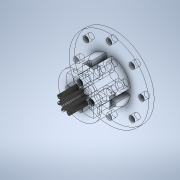
# Autodesk Inventor part: fixation_circle
Saved by Autodesk Inventor 2022.3 (Build 263350000, 350)
## iProperties
Created: 2022-01-31
Part Number: fixation_circle
Material: Generic
Document SubType Name: Modeling
Designer: Martijn
Density: 1 g/cm^3
Appearance: Default
Author: Martijn
Autodesk Inventor part; units mm, degrees
(part 1 of 2)
ref_plane "YZ Plane" through (0, 0, 0) normal (1, 0, 0) x (0, 1, 0)
ref_plane "XZ Plane" through (0, 0, 0) normal (0, 1, 0) x (-1, 0, 0)
ref_plane "XY Plane" through (0, 0, 0) normal (0, 0, 1) x (1, 0, 0)
sketch "Sketch1" plane through (0, 0, 0) normal (0, 0, 1) x (1, 0, 0)
  circle A0 centre (0, 0) radius 22
  circle A1 centre (0, 0) radius 2.6
  line L0 (-30.8, 0) -> (30.8, 0) projected
  line L1 (0, -30.8) -> (0, 30.8) projected
  dimension "d0" = 44
  dimension "d3" = 5.2
  dimension "d21" = 0
  constraints: 2 centre point, 2 coincident, 1 midpoint
  measures "d0" diameter of A0
  measures "d3" diameter of A1
  measures "d21" distance from line of L1 point (0, 0)
extrude "Extrusion1" add sketch "Sketch1" along normal blind 3 contours L0 A1 L1 A0 | A0 L1 A1 L0 | L1 A1 L0 A0 | A0 L0 A1 L1
sketch "Sketch3" plane through (0, 0, 3) normal (0, 0, 1) x (1, 0, 0)
  circle A0 centre (-18, 0) radius 1.6
  circle A1 centre (0, 0) radius 2.6 projected
  line L0 (-18, 0) -> (0, 0)
  line L1 (-63.2, 0) -> (36.2, 0) projected
  dimension "d11" = 3.2
  dimension "d12" = 18
  constraints: 2 end point, 1 centre point, 1 collinear
  measures "d11" diameter of A0
  measures "d12" distance of L0.end L0.start
extrude "Extrusion3" cut sketch "Sketch3" against normal blind 3 contours L0 L1 A0 | A0 L1 L0
pattern_circular "Circular Pattern2" count 8 over 360 about axis through (0, 0, 0) along (0, 0, 1) of "Extrusion3"
sketch "Sketch4" plane through (0, 0, 3) normal (0, 0, 1) x (1, 0, 0)
  circle A0 centre (0, 0) radius 12
  circle A1 centre (0, 0) radius 22 projected
  dimension "d20" = 24
  constraints: 1 centre point, 1 coincident, 1 concentric
  measures "d20" diameter of A0
extrude "Extrusion4" add sketch "Sketch4" along normal blind 16 contours A0
sketch "Sketch5" plane through (0, 0, 19) normal (0, 0, 1) x (1, 0, 0)
  line L0 (-2.1906, -4.3944) -> (-2.2181, -4.2687)
  line L1 (-2.2181, -4.2687) -> (-2.2394, -4.1474)
  line L2 (-2.2394, -4.1474) -> (-2.2546, -4.0331)
  line L3 (-2.2546, -4.0331) -> (-2.2645, -3.9235)
  line L4 (-2.2645, -3.9235) -> (-2.2694, -3.8217)
  line L5 (-2.2694, -3.8217) -> (-2.27, -3.7256)
  line L6 (-2.27, -3.7256) -> (-2.2668, -3.6359)
  line L7 (-2.2668, -3.6359) -> (-2.2603, -3.5527)
  line L8 (-2.2603, -3.5527) -> (-2.2403, -3.41)
  line L9 (-2.2403, -3.41) -> (-2.2136, -3.292)
  line L10 (-2.2136, -3.292) -> (-2.1861, -3.2049)
  line L11 (-2.1861, -3.2049) -> (-2.1603, -3.1417)
  line L12 (-2.1603, -3.1417) -> (-2.089, -3.0789)
  line L13 (-2.089, -3.0789) -> (-2.0175, -3.007)
  line L14 (-2.0175, -3.007) -> (-1.9555, -2.9347)
  line L15 (-1.9555, -2.9347) -> (-1.9031, -2.8628)
  line L16 (-1.9031, -2.8628) -> (-1.8599, -2.7919)
  line L17 (-1.8599, -2.7919) -> (-1.8259, -2.7226)
  line L18 (-1.8259, -2.7226) -> (-1.8008, -2.6557)
  line L19 (-1.8008, -2.6557) -> (-1.7844, -2.5917)
  line L20 (-1.7844, -2.5917) -> (-1.7763, -2.5312)
  line L21 (-1.7763, -2.5312) -> (-1.7762, -2.4748)
  line L22 (-1.7762, -2.4748) -> (-1.7838, -2.4231)
  line L23 (-1.7838, -2.4231) -> (-1.7986, -2.3766)
  line L24 (-1.7986, -2.3766) -> (-1.8203, -2.3358)
  line L25 (-1.8203, -2.3358) -> (-1.8522, -2.2972)
  line L26 (-1.8522, -2.2972) -> (-2.0138, -2.1559)
  line L27 (-2.0138, -2.1559) -> (-2.0861, -2.086)
  line L28 (-2.0861, -2.086) -> (-2.1559, -2.0138)
  line L29 (-2.1559, -2.0138) -> (-2.2973, -1.8521)
  line L30 (-2.2973, -1.8521) -> (-2.3358, -1.8202)
  line L31 (-2.3358, -1.8202) -> (-2.3766, -1.7986)
  line L32 (-2.3766, -1.7986) -> (-2.4232, -1.7838)
  line L33 (-2.4232, -1.7838) -> (-2.4749, -1.7762)
  line L34 (-2.4749, -1.7762) -> (-2.5313, -1.7763)
  line L35 (-2.5313, -1.7763) -> (-2.5917, -1.7843)
  line L36 (-2.5917, -1.7843) -> (-2.6557, -1.8008)
  line L37 (-2.6557, -1.8008) -> (-2.7227, -1.8259)
  line L38 (-2.7227, -1.8259) -> (-2.7919, -1.8599)
  line L39 (-2.7919, -1.8599) -> (-2.8628, -1.903)
  line L40 (-2.8628, -1.903) -> (-2.9347, -1.9555)
  line L41 (-2.9347, -1.9555) -> (-3.007, -2.0174)
  line L42 (-3.007, -2.0174) -> (-3.079, -2.089)
  line L43 (-3.079, -2.089) -> (-3.1417, -2.1602)
  line L44 (-3.1417, -2.1602) -> (-3.205, -2.1861)
  line L45 (-3.205, -2.1861) -> (-3.292, -2.2136)
  line L46 (-3.292, -2.2136) -> (-3.4101, -2.2403)
  line L47 (-3.4101, -2.2403) -> (-3.5527, -2.2603)
  line L48 (-3.5527, -2.2603) -> (-3.6359, -2.2668)
  line L49 (-3.6359, -2.2668) -> (-3.7257, -2.27)
  line L50 (-3.7257, -2.27) -> (-3.8217, -2.2694)
  line L51 (-3.8217, -2.2694) -> (-3.9235, -2.2644)
  line L52 (-3.9235, -2.2644) -> (-4.0331, -2.2546)
  line L53 (-4.0331, -2.2546) -> (-4.1474, -2.2394)
  line L54 (-4.1474, -2.2394) -> (-4.2688, -2.2181)
  line L55 (-4.2688, -2.2181) -> (-4.3944, -2.1905)
  line L56 (-4.3944, -2.1905) -> (-4.5093, -2.1604)
  arc A0 (-4.7162, -1.6609) -> (-4.5093, -2.1604) centre (-0.0001, -0.0001) ccw
  line L57 (-4.7162, -1.6609) -> (-4.6562, -1.5584)
  line L58 (-4.6562, -1.5584) -> (-4.5869, -1.4501)
  line L59 (-4.5869, -1.4501) -> (-4.5162, -1.3492)
  line L60 (-4.5162, -1.3492) -> (-4.4461, -1.2577)
  line L61 (-4.4461, -1.2577) -> (-4.3755, -1.1732)
  line L62 (-4.3755, -1.1732) -> (-4.307, -1.0977)
  line L63 (-4.307, -1.0977) -> (-4.2395, -1.0294)
  line L64 (-4.2395, -1.0294) -> (-4.1738, -0.9682)
  line L65 (-4.1738, -0.9682) -> (-4.1104, -0.914)
  line L66 (-4.1104, -0.914) -> (-3.9954, -0.8272)
  line L67 (-3.9954, -0.8272) -> (-3.893, -0.7626)
  line L68 (-3.893, -0.7626) -> (-3.812, -0.7205)
  line L69 (-3.812, -0.7205) -> (-3.749, -0.6941)
  line L70 (-3.749, -0.6941) -> (-3.6543, -0.7001)
  line L71 (-3.6543, -0.7001) -> (-3.5528, -0.6998)
  line L72 (-3.5528, -0.6998) -> (-3.4579, -0.6925)
  line L73 (-3.4579, -0.6925) -> (-3.3699, -0.6787)
  line L74 (-3.3699, -0.6787) -> (-3.2893, -0.6591)
  line L75 (-3.2893, -0.6591) -> (-3.2163, -0.6342)
  line L76 (-3.2163, -0.6342) -> (-3.1512, -0.6046)
  line L77 (-3.1512, -0.6046) -> (-3.0943, -0.571)
  line L78 (-3.0943, -0.571) -> (-3.0459, -0.5339)
  line L79 (-3.0459, -0.5339) -> (-3.0059, -0.4941)
  line L80 (-3.0059, -0.4941) -> (-2.9747, -0.4522)
  line L81 (-2.9747, -0.4522) -> (-2.9523, -0.4088)
  line L82 (-2.9523, -0.4088) -> (-2.9387, -0.3646)
  line L83 (-2.9387, -0.3646) -> (-2.9341, -0.3148)
  line L84 (-2.9341, -0.3148) -> (-2.9484, -0.1006)
  line L85 (-2.9484, -0.1006) -> (-2.9501, -0.0001)
  line L86 (-2.9501, -0.0001) -> (-2.9484, 0.1004)
  line L87 (-2.9484, 0.1004) -> (-2.9341, 0.3147)
  line L88 (-2.9341, 0.3147) -> (-2.9387, 0.3645)
  line L89 (-2.9387, 0.3645) -> (-2.9523, 0.4086)
  line L90 (-2.9523, 0.4086) -> (-2.9747, 0.452)
  line L91 (-2.9747, 0.452) -> (-3.0059, 0.494)
  line L92 (-3.0059, 0.494) -> (-3.0459, 0.5338)
  line L93 (-3.0459, 0.5338) -> (-3.0943, 0.5708)
  line L94 (-3.0943, 0.5708) -> (-3.1512, 0.6044)
  line L95 (-3.1512, 0.6044) -> (-3.2163, 0.634)
  line L96 (-3.2163, 0.634) -> (-3.2893, 0.6589)
  line L97 (-3.2893, 0.6589) -> (-3.3699, 0.6786)
  line L98 (-3.3699, 0.6786) -> (-3.4579, 0.6923)
  line L99 (-3.4579, 0.6923) -> (-3.5528, 0.6996)
  line L100 (-3.5528, 0.6996) -> (-3.6543, 0.6999)
  line L101 (-3.6543, 0.6999) -> (-3.749, 0.6939)
  line L102 (-3.749, 0.6939) -> (-3.812, 0.7203)
  line L103 (-3.812, 0.7203) -> (-3.893, 0.7625)
  line L104 (-3.893, 0.7625) -> (-3.9954, 0.8271)
  line L105 (-3.9954, 0.8271) -> (-4.1104, 0.9138)
  line L106 (-4.1104, 0.9138) -> (-4.1738, 0.968)
  line L107 (-4.1738, 0.968) -> (-4.2395, 1.0292)
  line L108 (-4.2395, 1.0292) -> (-4.307, 1.0976)
  line L109 (-4.307, 1.0976) -> (-4.3755, 1.173)
  line L110 (-4.3755, 1.173) -> (-4.4461, 1.2575)
  line L111 (-4.4461, 1.2575) -> (-4.5162, 1.3491)
  line L112 (-4.5162, 1.3491) -> (-4.5869, 1.4499)
  line L113 (-4.5869, 1.4499) -> (-4.6562, 1.5583)
  line L114 (-4.6562, 1.5583) -> (-4.7162, 1.6608)
  arc A1 (-4.5093, 2.1603) -> (-4.7162, 1.6608) centre (-0.0001, -0.0001) ccw
  line L115 (-4.5093, 2.1603) -> (-4.3944, 2.1904)
  line L116 (-4.3944, 2.1904) -> (-4.2688, 2.2179)
  line L117 (-4.2688, 2.2179) -> (-4.1474, 2.2392)
  line L118 (-4.1474, 2.2392) -> (-4.0331, 2.2544)
  line L119 (-4.0331, 2.2544) -> (-3.9235, 2.2643)
  line L120 (-3.9235, 2.2643) -> (-3.8217, 2.2692)
  line L121 (-3.8217, 2.2692) -> (-3.7257, 2.2698)
  line L122 (-3.7257, 2.2698) -> (-3.6359, 2.2666)
  line L123 (-3.6359, 2.2666) -> (-3.5527, 2.2601)
  line L124 (-3.5527, 2.2601) -> (-3.4101, 2.2401)
  line L125 (-3.4101, 2.2401) -> (-3.292, 2.2134)
  line L126 (-3.292, 2.2134) -> (-3.205, 2.186)
  line L127 (-3.205, 2.186) -> (-3.1417, 2.1601)
  line L128 (-3.1417, 2.1601) -> (-3.079, 2.0888)
  line L129 (-3.079, 2.0888) -> (-3.007, 2.0173)
  line L130 (-3.007, 2.0173) -> (-2.9347, 1.9553)
  line L131 (-2.9347, 1.9553) -> (-2.8628, 1.9029)
  line L132 (-2.8628, 1.9029) -> (-2.7919, 1.8597)
  line L133 (-2.7919, 1.8597) -> (-2.7227, 1.8257)
  line L134 (-2.7227, 1.8257) -> (-2.6557, 1.8006)
  line L135 (-2.6557, 1.8006) -> (-2.5917, 1.7842)
  line L136 (-2.5917, 1.7842) -> (-2.5313, 1.7761)
  line L137 (-2.5313, 1.7761) -> (-2.4749, 1.776)
  line L138 (-2.4749, 1.776) -> (-2.4232, 1.7836)
  line L139 (-2.4232, 1.7836) -> (-2.3766, 1.7984)
  line L140 (-2.3766, 1.7984) -> (-2.3358, 1.8201)
  line L141 (-2.3358, 1.8201) -> (-2.2973, 1.852)
  line L142 (-2.2973, 1.852) -> (-2.1559, 2.0136)
  line L143 (-2.1559, 2.0136) -> (-2.0861, 2.0859)
  line L144 (-2.0861, 2.0859) -> (-2.0138, 2.1557)
  line L145 (-2.0138, 2.1557) -> (-1.8522, 2.2971)
  line L146 (-1.8522, 2.2971) -> (-1.8203, 2.3356)
  line L147 (-1.8203, 2.3356) -> (-1.7986, 2.3764)
  line L148 (-1.7986, 2.3764) -> (-1.7838, 2.423)
  line L149 (-1.7838, 2.423) -> (-1.7762, 2.4747)
  line L150 (-1.7762, 2.4747) -> (-1.7763, 2.5311)
  line L151 (-1.7763, 2.5311) -> (-1.7844, 2.5916)
  line L152 (-1.7844, 2.5916) -> (-1.8008, 2.6556)
  line L153 (-1.8008, 2.6556) -> (-1.8259, 2.7225)
  line L154 (-1.8259, 2.7225) -> (-1.8599, 2.7917)
  line L155 (-1.8599, 2.7917) -> (-1.9031, 2.8626)
  line L156 (-1.9031, 2.8626) -> (-1.9555, 2.9345)
  line L157 (-1.9555, 2.9345) -> (-2.0175, 3.0068)
  line L158 (-2.0175, 3.0068) -> (-2.089, 3.0788)
  line L159 (-2.089, 3.0788) -> (-2.1603, 3.1415)
  line L160 (-2.1603, 3.1415) -> (-2.1861, 3.2048)
  line L161 (-2.1861, 3.2048) -> (-2.2136, 3.2918)
  line L162 (-2.2136, 3.2918) -> (-2.2403, 3.4099)
  line L163 (-2.2403, 3.4099) -> (-2.2603, 3.5526)
  line L164 (-2.2603, 3.5526) -> (-2.2668, 3.6357)
  line L165 (-2.2668, 3.6357) -> (-2.27, 3.7255)
  line L166 (-2.27, 3.7255) -> (-2.2694, 3.8215)
  line L167 (-2.2694, 3.8215) -> (-2.2645, 3.9233)
  line L168 (-2.2645, 3.9233) -> (-2.2546, 4.0329)
  line L169 (-2.2546, 4.0329) -> (-2.2394, 4.1473)
  line L170 (-2.2394, 4.1473) -> (-2.2181, 4.2686)
  line L171 (-2.2181, 4.2686) -> (-2.1906, 4.3942)
  line L172 (-2.1906, 4.3942) -> (-2.1605, 4.5091)
  arc A2 (-1.661, 4.716) -> (-2.1605, 4.5091) centre (-0.0001, -0.0001) ccw
  line L173 (-1.661, 4.716) -> (-1.5584, 4.656)
  line L174 (-1.5584, 4.656) -> (-1.4501, 4.5867)
  line L175 (-1.4501, 4.5867) -> (-1.3493, 4.516)
  line L176 (-1.3493, 4.516) -> (-1.2577, 4.4459)
  line L177 (-1.2577, 4.4459) -> (-1.1732, 4.3753)
  line L178 (-1.1732, 4.3753) -> (-1.0978, 4.3068)
  line L179 (-1.0978, 4.3068) -> (-1.0294, 4.2393)
  line L180 (-1.0294, 4.2393) -> (-0.9682, 4.1736)
  line L181 (-0.9682, 4.1736) -> (-0.914, 4.1102)
  line L182 (-0.914, 4.1102) -> (-0.8272, 3.9952)
  line L183 (-0.8272, 3.9952) -> (-0.7627, 3.8928)
  line L184 (-0.7627, 3.8928) -> (-0.7205, 3.8119)
  line L185 (-0.7205, 3.8119) -> (-0.6941, 3.7488)
  line L186 (-0.6941, 3.7488) -> (-0.7001, 3.6541)
  line L187 (-0.7001, 3.6541) -> (-0.6998, 3.5526)
  line L188 (-0.6998, 3.5526) -> (-0.6925, 3.4577)
  line L189 (-0.6925, 3.4577) -> (-0.6788, 3.3697)
  line L190 (-0.6788, 3.3697) -> (-0.6591, 3.2891)
  line L191 (-0.6591, 3.2891) -> (-0.6342, 3.2161)
  line L192 (-0.6342, 3.2161) -> (-0.6046, 3.151)
  line L193 (-0.6046, 3.151) -> (-0.571, 3.0942)
  line L194 (-0.571, 3.0942) -> (-0.534, 3.0457)
  line L195 (-0.534, 3.0457) -> (-0.4941, 3.0057)
  line L196 (-0.4941, 3.0057) -> (-0.4522, 2.9745)
  line L197 (-0.4522, 2.9745) -> (-0.4088, 2.9521)
  line L198 (-0.4088, 2.9521) -> (-0.3647, 2.9385)
  line L199 (-0.3647, 2.9385) -> (-0.3149, 2.9339)
  line L200 (-0.3149, 2.9339) -> (-0.1006, 2.9482)
  line L201 (-0.1006, 2.9482) -> (-0.0001, 2.9499)
  line L202 (-0.0001, 2.9499) -> (0.1004, 2.9482)
  line L203 (0.1004, 2.9482) -> (0.3146, 2.9339)
  line L204 (0.3146, 2.9339) -> (0.3644, 2.9385)
  line L205 (0.3644, 2.9385) -> (0.4086, 2.9521)
  line L206 (0.4086, 2.9521) -> (0.452, 2.9745)
  line L207 (0.452, 2.9745) -> (0.4939, 3.0057)
  line L208 (0.4939, 3.0057) -> (0.5337, 3.0457)
  line L209 (0.5337, 3.0457) -> (0.5708, 3.0942)
  line L210 (0.5708, 3.0942) -> (0.6044, 3.151)
  line L211 (0.6044, 3.151) -> (0.634, 3.2161)
  line L212 (0.634, 3.2161) -> (0.6589, 3.2891)
  line L213 (0.6589, 3.2891) -> (0.6785, 3.3697)
  line L214 (0.6785, 3.3697) -> (0.6923, 3.4577)
  line L215 (0.6923, 3.4577) -> (0.6996, 3.5526)
  line L216 (0.6996, 3.5526) -> (0.6999, 3.6541)
  line L217 (0.6999, 3.6541) -> (0.6939, 3.7488)
  line L218 (0.6939, 3.7488) -> (0.7203, 3.8119)
  line L219 (0.7203, 3.8119) -> (0.7624, 3.8928)
  line L220 (0.7624, 3.8928) -> (0.827, 3.9952)
  line L221 (0.827, 3.9952) -> (0.9138, 4.1102)
  line L222 (0.9138, 4.1102) -> (0.968, 4.1736)
  line L223 (0.968, 4.1736) -> (1.0292, 4.2393)
  line L224 (1.0292, 4.2393) -> (1.0975, 4.3068)
  line L225 (1.0975, 4.3068) -> (1.173, 4.3753)
  line L226 (1.173, 4.3753) -> (1.2575, 4.4459)
  line L227 (1.2575, 4.4459) -> (1.3491, 4.516)
  line L228 (1.3491, 4.516) -> (1.4499, 4.5867)
  line L229 (1.4499, 4.5867) -> (1.5582, 4.656)
  line L230 (1.5582, 4.656) -> (1.6607, 4.716)
  arc A3 (2.1602, 4.5091) -> (1.6607, 4.716) centre (-0.0001, -0.0001) ccw
  line L231 (2.1602, 4.5091) -> (2.1904, 4.3942)
  line L232 (2.1904, 4.3942) -> (2.2179, 4.2686)
  line L233 (2.2179, 4.2686) -> (2.2392, 4.1473)
  line L234 (2.2392, 4.1473) -> (2.2544, 4.0329)
  line L235 (2.2544, 4.0329) -> (2.2643, 3.9233)
  line L236 (2.2643, 3.9233) -> (2.2692, 3.8215)
  line L237 (2.2692, 3.8215) -> (2.2698, 3.7255)
  line L238 (2.2698, 3.7255) -> (2.2666, 3.6357)
  line L239 (2.2666, 3.6357) -> (2.2601, 3.5526)
  line L240 (2.2601, 3.5526) -> (2.2401, 3.4099)
  line L241 (2.2401, 3.4099) -> (2.2134, 3.2918)
  line L242 (2.2134, 3.2918) -> (2.1859, 3.2048)
  line L243 (2.1859, 3.2048) -> (2.16, 3.1415)
  line L244 (2.16, 3.1415) -> (2.0888, 3.0788)
  line L245 (2.0888, 3.0788) -> (2.0173, 3.0068)
  line L246 (2.0173, 3.0068) -> (1.9553, 2.9345)
  line L247 (1.9553, 2.9345) -> (1.9028, 2.8626)
  line L248 (1.9028, 2.8626) -> (1.8597, 2.7917)
  line L249 (1.8597, 2.7917) -> (1.8257, 2.7225)
  line L250 (1.8257, 2.7225) -> (1.8006, 2.6556)
  line L251 (1.8006, 2.6556) -> (1.7842, 2.5916)
  line L252 (1.7842, 2.5916) -> (1.7761, 2.5311)
  line L253 (1.7761, 2.5311) -> (1.776, 2.4747)
  line L254 (1.776, 2.4747) -> (1.7836, 2.423)
  line L255 (1.7836, 2.423) -> (1.7984, 2.3764)
  line L256 (1.7984, 2.3764) -> (1.82, 2.3356)
  line L257 (1.82, 2.3356) -> (1.8519, 2.2971)
  line L258 (1.8519, 2.2971) -> (2.0136, 2.1557)
  line L259 (2.0136, 2.1557) -> (2.0859, 2.0859)
  line L260 (2.0859, 2.0859) -> (2.1557, 2.0136)
  line L261 (2.1557, 2.0136) -> (2.2971, 1.852)
  line L262 (2.2971, 1.852) -> (2.3356, 1.8201)
  line L263 (2.3356, 1.8201) -> (2.3764, 1.7984)
  line L264 (2.3764, 1.7984) -> (2.4229, 1.7836)
  line L265 (2.4229, 1.7836) -> (2.4747, 1.776)
  line L266 (2.4747, 1.776) -> (2.531, 1.7761)
  line L267 (2.531, 1.7761) -> (2.5915, 1.7842)
  line L268 (2.5915, 1.7842) -> (2.6555, 1.8006)
  line L269 (2.6555, 1.8006) -> (2.7225, 1.8257)
  line L270 (2.7225, 1.8257) -> (2.7917, 1.8597)
  line L271 (2.7917, 1.8597) -> (2.8626, 1.9029)
  line L272 (2.8626, 1.9029) -> (2.9345, 1.9553)
  line L273 (2.9345, 1.9553) -> (3.0068, 2.0173)
  line L274 (3.0068, 2.0173) -> (3.0787, 2.0888)
  line L275 (3.0787, 2.0888) -> (3.1415, 2.1601)
  line L276 (3.1415, 2.1601) -> (3.2047, 2.186)
  line L277 (3.2047, 2.186) -> (3.2918, 2.2134)
  line L278 (3.2918, 2.2134) -> (3.4098, 2.2401)
  line L279 (3.4098, 2.2401) -> (3.5525, 2.2601)
  line L280 (3.5525, 2.2601) -> (3.6357, 2.2666)
  line L281 (3.6357, 2.2666) -> (3.7254, 2.2698)
  line L282 (3.7254, 2.2698) -> (3.8215, 2.2692)
  line L283 (3.8215, 2.2692) -> (3.9233, 2.2643)
  line L284 (3.9233, 2.2643) -> (4.0329, 2.2544)
  line L285 (4.0329, 2.2544) -> (4.1472, 2.2392)
  line L286 (4.1472, 2.2392) -> (4.2685, 2.2179)
  line L287 (4.2685, 2.2179) -> (4.3942, 2.1904)
  line L288 (4.3942, 2.1904) -> (4.509, 2.1603)
  arc A4 (4.7159, 1.6608) -> (4.509, 2.1603) centre (-0.0002, -0.0001) ccw
  line L289 (4.7159, 1.6608) -> (4.656, 1.5583)
  line L290 (4.656, 1.5583) -> (4.5866, 1.4499)
  line L291 (4.5866, 1.4499) -> (4.5159, 1.3491)
  line L292 (4.5159, 1.3491) -> (4.4458, 1.2575)
  line L293 (4.4458, 1.2575) -> (4.3753, 1.173)
  line L294 (4.3753, 1.173) -> (4.3068, 1.0976)
  line L295 (4.3068, 1.0976) -> (4.2393, 1.0292)
  line L296 (4.2393, 1.0292) -> (4.1736, 0.968)
  line L297 (4.1736, 0.968) -> (4.1102, 0.9138)
  line L298 (4.1102, 0.9138) -> (3.9952, 0.8271)
  line L299 (3.9952, 0.8271) -> (3.8928, 0.7625)
  line L300 (3.8928, 0.7625) -> (3.8118, 0.7203)
  line L301 (3.8118, 0.7203) -> (3.7488, 0.6939)
  line L302 (3.7488, 0.6939) -> (3.654, 0.6999)
  line L303 (3.654, 0.6999) -> (3.5526, 0.6996)
  line L304 (3.5526, 0.6996) -> (3.4577, 0.6923)
  line L305 (3.4577, 0.6923) -> (3.3697, 0.6786)
  line L306 (3.3697, 0.6786) -> (3.2891, 0.6589)
  line L307 (3.2891, 0.6589) -> (3.2161, 0.634)
  line L308 (3.2161, 0.634) -> (3.151, 0.6044)
  line L309 (3.151, 0.6044) -> (3.0941, 0.5708)
  line L310 (3.0941, 0.5708) -> (3.0456, 0.5338)
  line L311 (3.0456, 0.5338) -> (3.0057, 0.494)
  line L312 (3.0057, 0.494) -> (2.9745, 0.452)
  line L313 (2.9745, 0.452) -> (2.9521, 0.4086)
  line L314 (2.9521, 0.4086) -> (2.9385, 0.3645)
  line L315 (2.9385, 0.3645) -> (2.9338, 0.3147)
  line L316 (2.9338, 0.3147) -> (2.9482, 0.1004)
  line L317 (2.9482, 0.1004) -> (2.9499, -0.0001)
  line L318 (2.9499, -0.0001) -> (2.9482, -0.1006)
  line L319 (2.9482, -0.1006) -> (2.9338, -0.3148)
  line L320 (2.9338, -0.3148) -> (2.9385, -0.3646)
  line L321 (2.9385, -0.3646) -> (2.9521, -0.4088)
  line L322 (2.9521, -0.4088) -> (2.9745, -0.4522)
  line L323 (2.9745, -0.4522) -> (3.0057, -0.4941)
  line L324 (3.0057, -0.4941) -> (3.0456, -0.5339)
  line L325 (3.0456, -0.5339) -> (3.0941, -0.571)
  line L326 (3.0941, -0.571) -> (3.151, -0.6046)
  line L327 (3.151, -0.6046) -> (3.2161, -0.6342)
  line L328 (3.2161, -0.6342) -> (3.2891, -0.6591)
  line L329 (3.2891, -0.6591) -> (3.3697, -0.6787)
  line L330 (3.3697, -0.6787) -> (3.4577, -0.6925)
  line L331 (3.4577, -0.6925) -> (3.5526, -0.6998)
  line L332 (3.5526, -0.6998) -> (3.654, -0.7001)
  line L333 (3.654, -0.7001) -> (3.7488, -0.6941)
  line L334 (3.7488, -0.6941) -> (3.8118, -0.7205)
  line L335 (3.8118, -0.7205) -> (3.8928, -0.7626)
  line L336 (3.8928, -0.7626) -> (3.9952, -0.8272)
  line L337 (3.9952, -0.8272) -> (4.1102, -0.914)
  line L338 (4.1102, -0.914) -> (4.1736, -0.9682)
  line L339 (4.1736, -0.9682) -> (4.2393, -1.0294)
  line L340 (4.2393, -1.0294) -> (4.3068, -1.0977)
  line L341 (4.3068, -1.0977) -> (4.3753, -1.1732)
  line L342 (4.3753, -1.1732) -> (4.4458, -1.2577)
  line L343 (4.4458, -1.2577) -> (4.5159, -1.3492)
  line L344 (4.5159, -1.3492) -> (4.5866, -1.4501)
  line L345 (4.5866, -1.4501) -> (4.656, -1.5584)
  line L346 (4.656, -1.5584) -> (4.7159, -1.6609)
  arc A5 (4.509, -2.1604) -> (4.7159, -1.6609) centre (-0.0002, -0.0001) ccw
  line L347 (4.509, -2.1604) -> (4.3942, -2.1905)
  line L348 (4.3942, -2.1905) -> (4.2685, -2.2181)
  line L349 (4.2685, -2.2181) -> (4.1472, -2.2394)
  line L350 (4.1472, -2.2394) -> (4.0329, -2.2546)
  line L351 (4.0329, -2.2546) -> (3.9233, -2.2644)
  line L352 (3.9233, -2.2644) -> (3.8215, -2.2694)
  line L353 (3.8215, -2.2694) -> (3.7254, -2.27)
  line L354 (3.7254, -2.27) -> (3.6357, -2.2668)
  line L355 (3.6357, -2.2668) -> (3.5525, -2.2603)
  line L356 (3.5525, -2.2603) -> (3.4098, -2.2403)
  line L357 (3.4098, -2.2403) -> (3.2918, -2.2136)
  line L358 (3.2918, -2.2136) -> (3.2047, -2.1861)
  line L359 (3.2047, -2.1861) -> (3.1415, -2.1602)
  line L360 (3.1415, -2.1602) -> (3.0787, -2.089)
  line L361 (3.0787, -2.089) -> (3.0068, -2.0174)
  line L362 (3.0068, -2.0174) -> (2.9345, -1.9555)
  line L363 (2.9345, -1.9555) -> (2.8626, -1.903)
  line L364 (2.8626, -1.903) -> (2.7917, -1.8599)
  line L365 (2.7917, -1.8599) -> (2.7225, -1.8259)
  line L366 (2.7225, -1.8259) -> (2.6555, -1.8008)
  line L367 (2.6555, -1.8008) -> (2.5915, -1.7843)
  line L368 (2.5915, -1.7843) -> (2.531, -1.7763)
  line L369 (2.531, -1.7763) -> (2.4747, -1.7762)
  line L370 (2.4747, -1.7762) -> (2.4229, -1.7838)
  line L371 (2.4229, -1.7838) -> (2.3764, -1.7986)
  line L372 (2.3764, -1.7986) -> (2.3356, -1.8202)
  line L373 (2.3356, -1.8202) -> (2.2971, -1.8521)
  line L374 (2.2971, -1.8521) -> (2.1557, -2.0138)
  line L375 (2.1557, -2.0138) -> (2.0859, -2.086)
  line L376 (2.0859, -2.086) -> (2.0136, -2.1559)
  line L377 (2.0136, -2.1559) -> (1.8519, -2.2972)
  line L378 (1.8519, -2.2972) -> (1.82, -2.3358)
  line L379 (1.82, -2.3358) -> (1.7984, -2.3766)
  line L380 (1.7984, -2.3766) -> (1.7836, -2.4231)
  line L381 (1.7836, -2.4231) -> (1.776, -2.4748)
  line L382 (1.776, -2.4748) -> (1.7761, -2.5312)
  line L383 (1.7761, -2.5312) -> (1.7842, -2.5917)
  line L384 (1.7842, -2.5917) -> (1.8006, -2.6557)
  line L385 (1.8006, -2.6557) -> (1.8257, -2.7226)
  line L386 (1.8257, -2.7226) -> (1.8597, -2.7919)
  line L387 (1.8597, -2.7919) -> (1.9028, -2.8628)
  line L388 (1.9028, -2.8628) -> (1.9553, -2.9347)
  line L389 (1.9553, -2.9347) -> (2.0173, -3.007)
  line L390 (2.0173, -3.007) -> (2.0888, -3.0789)
  line L391 (2.0888, -3.0789) -> (2.16, -3.1417)
  line L392 (2.16, -3.1417) -> (2.1859, -3.2049)
  line L393 (2.1859, -3.2049) -> (2.2134, -3.292)
  line L394 (2.2134, -3.292) -> (2.2401, -3.41)
  line L395 (2.2401, -3.41) -> (2.2601, -3.5527)
  line L396 (2.2601, -3.5527) -> (2.2666, -3.6359)
  line L397 (2.2666, -3.6359) -> (2.2698, -3.7256)
  line L398 (2.2698, -3.7256) -> (2.2692, -3.8217)
  line L399 (2.2692, -3.8217) -> (2.2643, -3.9235)
  line L400 (2.2643, -3.9235) -> (2.2544, -4.0331)
  line L401 (2.2544, -4.0331) -> (2.2392, -4.1474)
  line L402 (2.2392, -4.1474) -> (2.2179, -4.2687)
  line L403 (2.2179, -4.2687) -> (2.1904, -4.3944)
  line L404 (2.1904, -4.3944) -> (2.1602, -4.5092)
  arc A6 (1.6607, -4.7161) -> (2.1602, -4.5092) centre (-0.0001, 0) ccw
  line L405 (1.6607, -4.7161) -> (1.5582, -4.6562)
  line L406 (1.5582, -4.6562) -> (1.4499, -4.5868)
  line L407 (1.4499, -4.5868) -> (1.3491, -4.5161)
  line L408 (1.3491, -4.5161) -> (1.2575, -4.446)
  line L409 (1.2575, -4.446) -> (1.173, -4.3755)
  line L410 (1.173, -4.3755) -> (1.0975, -4.307)
  line L411 (1.0975, -4.307) -> (1.0292, -4.2395)
  line L412 (1.0292, -4.2395) -> (0.968, -4.1738)
  line L413 (0.968, -4.1738) -> (0.9138, -4.1104)
  line L414 (0.9138, -4.1104) -> (0.827, -3.9954)
  line L415 (0.827, -3.9954) -> (0.7624, -3.893)
  line L416 (0.7624, -3.893) -> (0.7203, -3.812)
  line L417 (0.7203, -3.812) -> (0.6939, -3.749)
  line L418 (0.6939, -3.749) -> (0.6999, -3.6542)
  line L419 (0.6999, -3.6542) -> (0.6996, -3.5528)
  line L420 (0.6996, -3.5528) -> (0.6923, -3.4579)
  line L421 (0.6923, -3.4579) -> (0.6785, -3.3699)
  line L422 (0.6785, -3.3699) -> (0.6589, -3.2893)
  line L423 (0.6589, -3.2893) -> (0.634, -3.2163)
  line L424 (0.634, -3.2163) -> (0.6044, -3.1512)
  line L425 (0.6044, -3.1512) -> (0.5708, -3.0943)
  line L426 (0.5708, -3.0943) -> (0.5337, -3.0458)
  line L427 (0.5337, -3.0458) -> (0.4939, -3.0059)
  line L428 (0.4939, -3.0059) -> (0.452, -2.9747)
  line L429 (0.452, -2.9747) -> (0.4086, -2.9523)
  line L430 (0.4086, -2.9523) -> (0.3644, -2.9387)
  line L431 (0.3644, -2.9387) -> (0.3146, -2.934)
  line L432 (0.3146, -2.934) -> (0.1004, -2.9484)
  line L433 (0.1004, -2.9484) -> (-0.0001, -2.9501)
  line L434 (-0.0001, -2.9501) -> (-0.1006, -2.9484)
  line L435 (-0.1006, -2.9484) -> (-0.3149, -2.934)
  line L436 (-0.3149, -2.934) -> (-0.3647, -2.9387)
  line L437 (-0.3647, -2.9387) -> (-0.4088, -2.9523)
  line L438 (-0.4088, -2.9523) -> (-0.4522, -2.9747)
  line L439 (-0.4522, -2.9747) -> (-0.4941, -3.0059)
  line L440 (-0.4941, -3.0059) -> (-0.534, -3.0458)
  line L441 (-0.534, -3.0458) -> (-0.571, -3.0943)
  line L442 (-0.571, -3.0943) -> (-0.6046, -3.1512)
  line L443 (-0.6046, -3.1512) -> (-0.6342, -3.2163)
  line L444 (-0.6342, -3.2163) -> (-0.6591, -3.2893)
  line L445 (-0.6591, -3.2893) -> (-0.6788, -3.3699)
  line L446 (-0.6788, -3.3699) -> (-0.6925, -3.4579)
  line L447 (-0.6925, -3.4579) -> (-0.6998, -3.5528)
  line L448 (-0.6998, -3.5528) -> (-0.7001, -3.6542)
  line L449 (-0.7001, -3.6542) -> (-0.6941, -3.749)
  line L450 (-0.6941, -3.749) -> (-0.7205, -3.812)
  line L451 (-0.7205, -3.812) -> (-0.7627, -3.893)
  line L452 (-0.7627, -3.893) -> (-0.8272, -3.9954)
  line L453 (-0.8272, -3.9954) -> (-0.914, -4.1104)
  line L454 (-0.914, -4.1104) -> (-0.9682, -4.1738)
  line L455 (-0.9682, -4.1738) -> (-1.0294, -4.2395)
  line L456 (-1.0294, -4.2395) -> (-1.0978, -4.307)
  line L457 (-1.0978, -4.307) -> (-1.1732, -4.3755)
  line L458 (-1.1732, -4.3755) -> (-1.2577, -4.446)
  line L459 (-1.2577, -4.446) -> (-1.3493, -4.5161)
  line L460 (-1.3493, -4.5161) -> (-1.4501, -4.5868)
  line L461 (-1.4501, -4.5868) -> (-1.5584, -4.6562)
  line L462 (-1.5584, -4.6562) -> (-1.661, -4.7161)
  arc A7 (-2.1605, -4.5092) -> (-1.661, -4.7161) centre (-0.0001, 0) ccw
  line L463 (-2.1605, -4.5092) -> (-2.1906, -4.3944)
  line L464 (-3.3452, 2.6801) -> (-3.6666, 2.5292)
  line L465 (-3.6666, 2.5292) -> (-3.9743, 2.3925)
  line L466 (-3.9743, 2.3925) -> (-4.2682, 2.2692)
  line L467 (-4.2682, 2.2692) -> (-4.5472, 2.1589)
  line L468 (-4.5472, 2.1589) -> (-4.8121, 2.0607)
  line L469 (-4.8121, 2.0607) -> (-5.0226, 1.9866)
  line L470 (-5.0226, 1.9866) -> (-5.0656, 1.9647)
  line L471 (-5.0656, 1.9647) -> (-5.0795, 1.9535)
  line L472 (-5.0795, 1.9535) -> (-5.0884, 1.9423)
  line L473 (-5.0884, 1.9423) -> (-5.0922, 1.9312)
  line L474 (-5.0922, 1.9312) -> (-5.0901, 1.8783)
  line L475 (-5.0901, 1.8783) -> (-5.0769, 1.5338)
  line L476 (-5.0769, 1.5338) -> (-5.0661, 1.1891)
  line L477 (-5.0661, 1.1891) -> (-5.0645, 1.1362)
  line L478 (-5.0645, 1.1362) -> (-5.0599, 1.1254)
  line L479 (-5.0599, 1.1254) -> (-5.0502, 1.1148)
  line L480 (-5.0502, 1.1148) -> (-5.0356, 1.1046)
  line L481 (-5.0356, 1.1046) -> (-4.9911, 1.0858)
  line L482 (-4.9911, 1.0858) -> (-4.776, 1.0266)
  line L483 (-4.776, 1.0266) -> (-4.5049, 0.947)
  line L484 (-4.5049, 0.947) -> (-4.2189, 0.8566)
  line L485 (-4.2189, 0.8566) -> (-3.917, 0.7541)
  line L486 (-3.917, 0.7541) -> (-3.6006, 0.6392)
  line L487 (-3.6006, 0.6392) -> (-3.2695, 0.511)
  line L488 (-3.2695, 0.511) -> (-3.0019, 0.4017)
  arc A8 (-3.0019, -0.4018) -> (-3.0019, 0.4017) centre (-49.0001, -0.0001) ccw
  line L489 (-3.0019, -0.4018) -> (-3.2695, -0.5112)
  line L490 (-3.2695, -0.5112) -> (-3.6006, -0.6393)
  line L491 (-3.6006, -0.6393) -> (-3.917, -0.7542)
  line L492 (-3.917, -0.7542) -> (-4.2189, -0.8567)
  line L493 (-4.2189, -0.8567) -> (-4.5049, -0.9472)
  line L494 (-4.5049, -0.9472) -> (-4.776, -1.0268)
  line L495 (-4.776, -1.0268) -> (-4.9911, -1.086)
  line L496 (-4.9911, -1.086) -> (-5.0356, -1.1048)
  line L497 (-5.0356, -1.1048) -> (-5.0502, -1.115)
  line L498 (-5.0502, -1.115) -> (-5.0599, -1.1255)
  line L499 (-5.0599, -1.1255) -> (-5.0645, -1.1364)
  line L500 (-5.0645, -1.1364) -> (-5.0661, -1.1893)
  line L501 (-5.0661, -1.1893) -> (-5.0769, -1.5339)
  line L502 (-5.0769, -1.5339) -> (-5.0901, -1.8785)
  line L503 (-5.0901, -1.8785) -> (-5.0922, -1.9313)
  line L504 (-5.0922, -1.9313) -> (-5.0884, -1.9425)
  line L505 (-5.0884, -1.9425) -> (-5.0795, -1.9537)
  line L506 (-5.0795, -1.9537) -> (-5.0656, -1.9649)
  line L507 (-5.0656, -1.9649) -> (-5.0226, -1.9868)
  line L508 (-5.0226, -1.9868) -> (-4.8121, -2.0608)
  line L509 (-4.8121, -2.0608) -> (-4.5472, -2.1591)
  line L510 (-4.5472, -2.1591) -> (-4.2682, -2.2693)
  line L511 (-4.2682, -2.2693) -> (-3.9743, -2.3926)
  line L512 (-3.9743, -2.3926) -> (-3.6666, -2.5293)
  line L513 (-3.6666, -2.5293) -> (-3.3452, -2.6802)
  line L514 (-3.3452, -2.6802) -> (-3.0859, -2.808)
  arc A9 (-3.1419, -3.6095) -> (-3.0859, -2.808) centre (-49.0001, -0.0001) ccw
  line L515 (-3.1419, -3.6095) -> (-3.4165, -3.7)
  line L516 (-3.4165, -3.7) -> (-3.7558, -3.8047)
  line L517 (-3.7558, -3.8047) -> (-4.0795, -3.8972)
  line L518 (-4.0795, -3.8972) -> (-4.3877, -3.9784)
  line L519 (-4.3877, -3.9784) -> (-4.6793, -4.0487)
  line L520 (-4.6793, -4.0487) -> (-4.9553, -4.1092)
  line L521 (-4.9553, -4.1092) -> (-5.1741, -4.1532)
  line L522 (-5.1741, -4.1532) -> (-5.2197, -4.1689)
  line L523 (-5.2197, -4.1689) -> (-5.2351, -4.178)
  line L524 (-5.2351, -4.178) -> (-5.2454, -4.1879)
  line L525 (-5.2454, -4.1879) -> (-5.2508, -4.1984)
  line L526 (-5.2508, -4.1984) -> (-5.256, -4.2511)
  line L527 (-5.256, -4.2511) -> (-5.2909, -4.5941)
  line L528 (-5.2909, -4.5941) -> (-5.3281, -4.9369)
  line L529 (-5.3281, -4.9369) -> (-5.3339, -4.9895)
  line L530 (-5.3339, -4.9895) -> (-5.3309, -5.0009)
  line L531 (-5.3309, -5.0009) -> (-5.3228, -5.0127)
  line L532 (-5.3228, -5.0127) -> (-5.3097, -5.0248)
  line L533 (-5.3097, -5.0248) -> (-5.2683, -5.0496)
  line L534 (-5.2683, -5.0496) -> (-5.0635, -5.1382)
  line L535 (-5.0635, -5.1382) -> (-4.8061, -5.2547)
  line L536 (-4.8061, -5.2547) -> (-4.5355, -5.3841)
  line L537 (-4.8061, 5.2546) -> (-5.0635, 5.138)
  line L538 (-5.0635, 5.138) -> (-5.2683, 5.0495)
  line L539 (-5.2683, 5.0495) -> (-5.3097, 5.0247)
  line L540 (-5.3097, 5.0247) -> (-5.3228, 5.0125)
  line L541 (-5.3228, 5.0125) -> (-5.3309, 5.0007)
  line L542 (-5.3309, 5.0007) -> (-5.3339, 4.9893)
  line L543 (-5.3339, 4.9893) -> (-5.3281, 4.9367)
  line L544 (-5.3281, 4.9367) -> (-5.2909, 4.5939)
  line L545 (-5.2909, 4.5939) -> (-5.256, 4.2509)
  line L546 (-5.256, 4.2509) -> (-5.2508, 4.1982)
  line L547 (-5.2508, 4.1982) -> (-5.2454, 4.1878)
  line L548 (-5.2454, 4.1878) -> (-5.2351, 4.1779)
  line L549 (-5.2351, 4.1779) -> (-5.2197, 4.1687)
  line L550 (-5.2197, 4.1687) -> (-5.1741, 4.1531)
  line L551 (-5.1741, 4.1531) -> (-4.9553, 4.109)
  line L552 (-4.9553, 4.109) -> (-4.6793, 4.0486)
  line L553 (-4.6793, 4.0486) -> (-4.3877, 3.9783)
  line L554 (-4.3877, 3.9783) -> (-4.0795, 3.8971)
  line L555 (-4.0795, 3.8971) -> (-3.7558, 3.8045)
  line L556 (-3.7558, 3.8045) -> (-3.4165, 3.6998)
  line L557 (-3.4165, 3.6998) -> (-3.1419, 3.6094)
  arc A10 (-3.0859, 2.8078) -> (-3.1419, 3.6094) centre (-49.0001, -0.0001) ccw
  line L558 (-3.0859, 2.8078) -> (-3.3452, 2.6801)
  line L559 (-2.1906, -4.3944) -> (-2.2181, -4.2687)
  line L560 (-2.2181, -4.2687) -> (-2.2394, -4.1474)
  line L561 (-2.2394, -4.1474) -> (-2.2546, -4.0331)
  line L562 (-2.2546, -4.0331) -> (-2.2645, -3.9235)
  line L563 (-2.2645, -3.9235) -> (-2.2694, -3.8217)
  line L564 (-2.2694, -3.8217) -> (-2.27, -3.7256)
  line L565 (-2.27, -3.7256) -> (-2.2668, -3.6359)
  line L566 (-2.2668, -3.6359) -> (-2.2603, -3.5527)
  line L567 (-2.2603, -3.5527) -> (-2.2403, -3.41)
  line L568 (-2.2403, -3.41) -> (-2.2136, -3.292)
  line L569 (-2.2136, -3.292) -> (-2.1861, -3.2049)
  line L570 (-2.1861, -3.2049) -> (-2.1603, -3.1417)
  line L571 (-2.1603, -3.1417) -> (-2.089, -3.0789)
  line L572 (-2.089, -3.0789) -> (-2.0175, -3.007)
  line L573 (-2.0175, -3.007) -> (-1.9555, -2.9347)
  line L574 (-1.9555, -2.9347) -> (-1.9031, -2.8628)
  line L575 (-1.9031, -2.8628) -> (-1.8599, -2.7919)
  line L576 (-1.8599, -2.7919) -> (-1.8259, -2.7226)
  line L577 (-1.8259, -2.7226) -> (-1.8008, -2.6557)
  line L578 (-1.8008, -2.6557) -> (-1.7844, -2.5917)
  line L579 (-1.7844, -2.5917) -> (-1.7763, -2.5312)
  line L580 (-1.7763, -2.5312) -> (-1.7762, -2.4748)
  line L581 (-1.7762, -2.4748) -> (-1.7838, -2.4231)
  line L582 (-1.7838, -2.4231) -> (-1.7986, -2.3766)
  line L583 (-1.7986, -2.3766) -> (-1.8203, -2.3358)
  line L584 (-1.8203, -2.3358) -> (-1.8522, -2.2972)
  line L585 (-1.8522, -2.2972) -> (-2.0138, -2.1559)
  line L586 (-2.0138, -2.1559) -> (-2.0861, -2.086)
  line L587 (-2.0861, -2.086) -> (-2.1559, -2.0138)
  line L588 (-2.1559, -2.0138) -> (-2.2973, -1.8521)
  line L589 (-2.2973, -1.8521) -> (-2.3358, -1.8202)
  line L590 (-2.3358, -1.8202) -> (-2.3766, -1.7986)
  line L591 (-2.3766, -1.7986) -> (-2.4232, -1.7838)
  line L592 (-2.4232, -1.7838) -> (-2.4749, -1.7762)
  line L593 (-2.4749, -1.7762) -> (-2.5313, -1.7763)
  line L594 (-2.5313, -1.7763) -> (-2.5917, -1.7843)
  line L595 (-2.5917, -1.7843) -> (-2.6557, -1.8008)
  line L596 (-2.6557, -1.8008) -> (-2.7227, -1.8259)
  line L597 (-2.7227, -1.8259) -> (-2.7919, -1.8599)
  line L598 (-2.7919, -1.8599) -> (-2.8628, -1.903)
  line L599 (-2.8628, -1.903) -> (-2.9347, -1.9555)
  line L600 (-2.9347, -1.9555) -> (-3.007, -2.0174)
  line L601 (-3.007, -2.0174) -> (-3.079, -2.089)
  line L602 (-3.079, -2.089) -> (-3.1417, -2.1602)
  line L603 (-3.1417, -2.1602) -> (-3.205, -2.1861)
  line L604 (-3.205, -2.1861) -> (-3.292, -2.2136)
  line L605 (-3.292, -2.2136) -> (-3.4101, -2.2403)
  line L606 (-3.4101, -2.2403) -> (-3.5527, -2.2603)
  line L607 (-3.5527, -2.2603) -> (-3.6359, -2.2668)
  line L608 (-3.6359, -2.2668) -> (-3.7257, -2.27)
  line L609 (-3.7257, -2.27) -> (-3.8217, -2.2694)
  line L610 (-3.8217, -2.2694) -> (-3.9235, -2.2644)
  line L611 (-3.9235, -2.2644) -> (-4.0331, -2.2546)
  line L612 (-4.0331, -2.2546) -> (-4.1474, -2.2394)
  line L613 (-4.1474, -2.2394) -> (-4.2688, -2.2181)
  line L614 (-4.2688, -2.2181) -> (-4.3944, -2.1905)
  line L615 (-4.3944, -2.1905) -> (-4.5093, -2.1604)
  arc A11 (-4.7162, -1.6609) -> (-4.5093, -2.1604) centre (-0.0001, -0.0001) ccw
  line L616 (-4.7162, -1.6609) -> (-4.6562, -1.5584)
  line L617 (-4.6562, -1.5584) -> (-4.5869, -1.4501)
  line L618 (-4.5869, -1.4501) -> (-4.5162, -1.3492)
  line L619 (-4.5162, -1.3492) -> (-4.4461, -1.2577)
  line L620 (-4.4461, -1.2577) -> (-4.3755, -1.1732)
  line L621 (-4.3755, -1.1732) -> (-4.307, -1.0977)
  line L622 (-4.307, -1.0977) -> (-4.2395, -1.0294)
  line L623 (-4.2395, -1.0294) -> (-4.1738, -0.9682)
  line L624 (-4.1738, -0.9682) -> (-4.1104, -0.914)
  line L625 (-4.1104, -0.914) -> (-3.9954, -0.8272)
  line L626 (-3.9954, -0.8272) -> (-3.893, -0.7626)
  line L627 (-3.893, -0.7626) -> (-3.812, -0.7205)
  line L628 (-3.812, -0.7205) -> (-3.749, -0.6941)
  line L629 (-3.749, -0.6941) -> (-3.6543, -0.7001)
  line L630 (-3.6543, -0.7001) -> (-3.5528, -0.6998)
  line L631 (-3.5528, -0.6998) -> (-3.4579, -0.6925)
  line L632 (-3.4579, -0.6925) -> (-3.3699, -0.6787)
  line L633 (-3.3699, -0.6787) -> (-3.2893, -0.6591)
  line L634 (-3.2893, -0.6591) -> (-3.2163, -0.6342)
  line L635 (-3.2163, -0.6342) -> (-3.1512, -0.6046)
  line L636 (-3.1512, -0.6046) -> (-3.0943, -0.571)
  line L637 (-3.0943, -0.571) -> (-3.0459, -0.5339)
  line L638 (-3.0459, -0.5339) -> (-3.0059, -0.4941)
  line L639 (-3.0059, -0.4941) -> (-2.9747, -0.4522)
  line L640 (-2.9747, -0.4522) -> (-2.9523, -0.4088)
  line L641 (-2.9523, -0.4088) -> (-2.9387, -0.3646)
  line L642 (-2.9387, -0.3646) -> (-2.9341, -0.3148)
  line L643 (-2.9341, -0.3148) -> (-2.9484, -0.1006)
  line L644 (-2.9484, -0.1006) -> (-2.9501, -0.0001)
  line L645 (-2.9501, -0.0001) -> (-2.9484, 0.1004)
  line L646 (-2.9484, 0.1004) -> (-2.9341, 0.3147)
  line L647 (-2.9341, 0.3147) -> (-2.9387, 0.3645)
  line L648 (-2.9387, 0.3645) -> (-2.9523, 0.4086)
  line L649 (-2.9523, 0.4086) -> (-2.9747, 0.452)
  line L650 (-2.9747, 0.452) -> (-3.0059, 0.494)
  line L651 (-3.0059, 0.494) -> (-3.0459, 0.5338)
  line L652 (-3.0459, 0.5338) -> (-3.0943, 0.5708)
  line L653 (-3.0943, 0.5708) -> (-3.1512, 0.6044)
  line L654 (-3.1512, 0.6044) -> (-3.2163, 0.634)
  line L655 (-3.2163, 0.634) -> (-3.2893, 0.6589)
  line L656 (-3.2893, 0.6589) -> (-3.3699, 0.6786)
  line L657 (-3.3699, 0.6786) -> (-3.4579, 0.6923)
  line L658 (-3.4579, 0.6923) -> (-3.5528, 0.6996)
  line L659 (-3.5528, 0.6996) -> (-3.6543, 0.6999)
  line L660 (-3.6543, 0.6999) -> (-3.749, 0.6939)
  line L661 (-3.749, 0.6939) -> (-3.812, 0.7203)
  line L662 (-3.812, 0.7203) -> (-3.893, 0.7625)
  line L663 (-3.893, 0.7625) -> (-3.9954, 0.8271)
  line L664 (-3.9954, 0.8271) -> (-4.1104, 0.9138)
  line L665 (-4.1104, 0.9138) -> (-4.1738, 0.968)
  line L666 (-4.1738, 0.968) -> (-4.2395, 1.0292)
  line L667 (-4.2395, 1.0292) -> (-4.307, 1.0976)
  line L668 (-4.307, 1.0976) -> (-4.3755, 1.173)
  line L669 (-4.3755, 1.173) -> (-4.4461, 1.2575)
  line L670 (-4.4461, 1.2575) -> (-4.5162, 1.3491)
  line L671 (-4.5162, 1.3491) -> (-4.5869, 1.4499)
  line L672 (-4.5869, 1.4499) -> (-4.6562, 1.5583)
  line L673 (-4.6562, 1.5583) -> (-4.7162, 1.6608)
  arc A12 (-4.5093, 2.1603) -> (-4.7162, 1.6608) centre (-0.0001, -0.0001) ccw
  line L674 (-4.5093, 2.1603) -> (-4.3944, 2.1904)
  line L675 (-4.3944, 2.1904) -> (-4.2688, 2.2179)
  line L676 (-4.2688, 2.2179) -> (-4.1474, 2.2392)
  line L677 (-4.1474, 2.2392) -> (-4.0331, 2.2544)
  line L678 (-4.0331, 2.2544) -> (-3.9235, 2.2643)
  line L679 (-3.9235, 2.2643) -> (-3.8217, 2.2692)
  line L680 (-3.8217, 2.2692) -> (-3.7257, 2.2698)
  line L681 (-3.7257, 2.2698) -> (-3.6359, 2.2666)
  line L682 (-3.6359, 2.2666) -> (-3.5527, 2.2601)
  line L683 (-3.5527, 2.2601) -> (-3.4101, 2.2401)
  line L684 (-3.4101, 2.2401) -> (-3.292, 2.2134)
  line L685 (-3.292, 2.2134) -> (-3.205, 2.186)
  line L686 (-3.205, 2.186) -> (-3.1417, 2.1601)
  line L687 (-3.1417, 2.1601) -> (-3.079, 2.0888)
  line L688 (-3.079, 2.0888) -> (-3.007, 2.0173)
  line L689 (-3.007, 2.0173) -> (-2.9347, 1.9553)
  line L690 (-2.9347, 1.9553) -> (-2.8628, 1.9029)
  line L691 (-2.8628, 1.9029) -> (-2.7919, 1.8597)
  line L692 (-2.7919, 1.8597) -> (-2.7227, 1.8257)
  line L693 (-2.7227, 1.8257) -> (-2.6557, 1.8006)
  line L694 (-2.6557, 1.8006) -> (-2.5917, 1.7842)
  line L695 (-2.5917, 1.7842) -> (-2.5313, 1.7761)
  line L696 (-2.5313, 1.7761) -> (-2.4749, 1.776)
  line L697 (-2.4749, 1.776) -> (-2.4232, 1.7836)
  line L698 (-2.4232, 1.7836) -> (-2.3766, 1.7984)
  line L699 (-2.3766, 1.7984) -> (-2.3358, 1.8201)
  line L700 (-2.3358, 1.8201) -> (-2.2973, 1.852)
  line L701 (-2.2973, 1.852) -> (-2.1559, 2.0136)
  line L702 (-2.1559, 2.0136) -> (-2.0861, 2.0859)
  line L703 (-2.0861, 2.0859) -> (-2.0138, 2.1557)
  line L704 (-2.0138, 2.1557) -> (-1.8522, 2.2971)
  line L705 (-1.8522, 2.2971) -> (-1.8203, 2.3356)
  line L706 (-1.8203, 2.3356) -> (-1.7986, 2.3764)
  line L707 (-1.7986, 2.3764) -> (-1.7838, 2.423)
  line L708 (-1.7838, 2.423) -> (-1.7762, 2.4747)
  line L709 (-1.7762, 2.4747) -> (-1.7763, 2.5311)
  line L710 (-1.7763, 2.5311) -> (-1.7844, 2.5916)
  line L711 (-1.7844, 2.5916) -> (-1.8008, 2.6556)
  line L712 (-1.8008, 2.6556) -> (-1.8259, 2.7225)
  line L713 (-1.8259, 2.7225) -> (-1.8599, 2.7917)
  line L714 (-1.8599, 2.7917) -> (-1.9031, 2.8626)
  line L715 (-1.9031, 2.8626) -> (-1.9555, 2.9345)
  line L716 (-1.9555, 2.9345) -> (-2.0175, 3.0068)
  line L717 (-2.0175, 3.0068) -> (-2.089, 3.0788)
  line L718 (-2.089, 3.0788) -> (-2.1603, 3.1415)
  line L719 (-2.1603, 3.1415) -> (-2.1861, 3.2048)
  line L720 (-2.1861, 3.2048) -> (-2.2136, 3.2918)
  line L721 (-2.2136, 3.2918) -> (-2.2403, 3.4099)
  line L722 (-2.2403, 3.4099) -> (-2.2603, 3.5526)
  line L723 (-2.2603, 3.5526) -> (-2.2668, 3.6357)
  line L724 (-2.2668, 3.6357) -> (-2.27, 3.7255)
  line L725 (-2.27, 3.7255) -> (-2.2694, 3.8215)
  line L726 (-2.2694, 3.8215) -> (-2.2645, 3.9233)
  line L727 (-2.2645, 3.9233) -> (-2.2546, 4.0329)
  line L728 (-2.2546, 4.0329) -> (-2.2394, 4.1473)
  line L729 (-2.2394, 4.1473) -> (-2.2181, 4.2686)
  line L730 (-2.2181, 4.2686) -> (-2.1906, 4.3942)
  line L731 (-2.1906, 4.3942) -> (-2.1605, 4.5091)
  arc A13 (-1.661, 4.716) -> (-2.1605, 4.5091) centre (-0.0001, -0.0001) ccw
  line L732 (-1.661, 4.716) -> (-1.5584, 4.656)
  line L733 (-1.5584, 4.656) -> (-1.4501, 4.5867)
  line L734 (-1.4501, 4.5867) -> (-1.3493, 4.516)
  line L735 (-1.3493, 4.516) -> (-1.2577, 4.4459)
  line L736 (-1.2577, 4.4459) -> (-1.1732, 4.3753)
  line L737 (-1.1732, 4.3753) -> (-1.0978, 4.3068)
  line L738 (-1.0978, 4.3068) -> (-1.0294, 4.2393)
  line L739 (-1.0294, 4.2393) -> (-0.9682, 4.1736)
  line L740 (-0.9682, 4.1736) -> (-0.914, 4.1102)
  line L741 (-0.914, 4.1102) -> (-0.8272, 3.9952)
  line L742 (-0.8272, 3.9952) -> (-0.7627, 3.8928)
  line L743 (-0.7627, 3.8928) -> (-0.7205, 3.8119)
  line L744 (-0.7205, 3.8119) -> (-0.6941, 3.7488)
  line L745 (-0.6941, 3.7488) -> (-0.7001, 3.6541)
  line L746 (-0.7001, 3.6541) -> (-0.6998, 3.5526)
  line L747 (-0.6998, 3.5526) -> (-0.6925, 3.4577)
  line L748 (-0.6925, 3.4577) -> (-0.6788, 3.3697)
  line L749 (-0.6788, 3.3697) -> (-0.6591, 3.2891)
  line L750 (-0.6591, 3.2891) -> (-0.6342, 3.2161)
  line L751 (-0.6342, 3.2161) -> (-0.6046, 3.151)
  line L752 (-0.6046, 3.151) -> (-0.571, 3.0942)
  line L753 (-0.571, 3.0942) -> (-0.534, 3.0457)
  line L754 (-0.534, 3.0457) -> (-0.4941, 3.0057)
  line L755 (-0.4941, 3.0057) -> (-0.4522, 2.9745)
  line L756 (-0.4522, 2.9745) -> (-0.4088, 2.9521)
  line L757 (-0.4088, 2.9521) -> (-0.3647, 2.9385)
  line L758 (-0.3647, 2.9385) -> (-0.3149, 2.9339)
  line L759 (-0.3149, 2.9339) -> (-0.1006, 2.9482)
  line L760 (-0.1006, 2.9482) -> (-0.0001, 2.9499)
  line L761 (-0.0001, 2.9499) -> (0.1004, 2.9482)
  line L762 (0.1004, 2.9482) -> (0.3146, 2.9339)
  line L763 (0.3146, 2.9339) -> (0.3644, 2.9385)
  line L764 (0.3644, 2.9385) -> (0.4086, 2.9521)
  line L765 (0.4086, 2.9521) -> (0.452, 2.9745)
  line L766 (0.452, 2.9745) -> (0.4939, 3.0057)
  line L767 (0.4939, 3.0057) -> (0.5337, 3.0457)
  line L768 (0.5337, 3.0457) -> (0.5708, 3.0942)
  line L769 (0.5708, 3.0942) -> (0.6044, 3.151)
  line L770 (0.6044, 3.151) -> (0.634, 3.2161)
  line L771 (0.634, 3.2161) -> (0.6589, 3.2891)
  line L772 (0.6589, 3.2891) -> (0.6785, 3.3697)
  line L773 (0.6785, 3.3697) -> (0.6923, 3.4577)
  line L774 (0.6923, 3.4577) -> (0.6996, 3.5526)
  line L775 (0.6996, 3.5526) -> (0.6999, 3.6541)
  line L776 (0.6999, 3.6541) -> (0.6939, 3.7488)
  line L777 (0.6939, 3.7488) -> (0.7203, 3.8119)
  line L778 (0.7203, 3.8119) -> (0.7624, 3.8928)
  line L779 (0.7624, 3.8928) -> (0.827, 3.9952)
  line L780 (0.827, 3.9952) -> (0.9138, 4.1102)
  line L781 (0.9138, 4.1102) -> (0.968, 4.1736)
  line L782 (0.968, 4.1736) -> (1.0292, 4.2393)
  line L783 (1.0292, 4.2393) -> (1.0975, 4.3068)
  line L784 (1.0975, 4.3068) -> (1.173, 4.3753)
  line L785 (1.173, 4.3753) -> (1.2575, 4.4459)
  line L786 (1.2575, 4.4459) -> (1.3491, 4.516)
  line L787 (1.3491, 4.516) -> (1.4499, 4.5867)
  line L788 (1.4499, 4.5867) -> (1.5582, 4.656)
  line L789 (1.5582, 4.656) -> (1.6607, 4.716)
  arc A14 (2.1602, 4.5091) -> (1.6607, 4.716) centre (-0.0001, -0.0001) ccw
  line L790 (2.1602, 4.5091) -> (2.1904, 4.3942)
  line L791 (2.1904, 4.3942) -> (2.2179, 4.2686)
  line L792 (2.2179, 4.2686) -> (2.2392, 4.1473)
  line L793 (2.2392, 4.1473) -> (2.2544, 4.0329)
  line L794 (2.2544, 4.0329) -> (2.2643, 3.9233)
  line L795 (2.2643, 3.9233) -> (2.2692, 3.8215)
  line L796 (2.2692, 3.8215) -> (2.2698, 3.7255)
  line L797 (2.2698, 3.7255) -> (2.2666, 3.6357)
  line L798 (2.2666, 3.6357) -> (2.2601, 3.5526)
  line L799 (2.2601, 3.5526) -> (2.2401, 3.4099)
  line L800 (2.2401, 3.4099) -> (2.2134, 3.2918)
  line L801 (2.2134, 3.2918) -> (2.1859, 3.2048)
  line L802 (2.1859, 3.2048) -> (2.16, 3.1415)
  line L803 (2.16, 3.1415) -> (2.0888, 3.0788)
  line L804 (2.0888, 3.0788) -> (2.0173, 3.0068)
  line L805 (2.0173, 3.0068) -> (1.9553, 2.9345)
  line L806 (1.9553, 2.9345) -> (1.9028, 2.8626)
  line L807 (1.9028, 2.8626) -> (1.8597, 2.7917)
  line L808 (1.8597, 2.7917) -> (1.8257, 2.7225)
  line L809 (1.8257, 2.7225) -> (1.8006, 2.6556)
  line L810 (1.8006, 2.6556) -> (1.7842, 2.5916)
  line L811 (1.7842, 2.5916) -> (1.7761, 2.5311)
  line L812 (1.7761, 2.5311) -> (1.776, 2.4747)
  line L813 (1.776, 2.4747) -> (1.7836, 2.423)
  line L814 (1.7836, 2.423) -> (1.7984, 2.3764)
  line L815 (1.7984, 2.3764) -> (1.82, 2.3356)
  line L816 (1.82, 2.3356) -> (1.8519, 2.2971)
  line L817 (1.8519, 2.2971) -> (2.0136, 2.1557)
  line L818 (2.0136, 2.1557) -> (2.0859, 2.0859)
  line L819 (2.0859, 2.0859) -> (2.1557, 2.0136)
  line L820 (2.1557, 2.0136) -> (2.2971, 1.852)
  line L821 (2.2971, 1.852) -> (2.3356, 1.8201)
  line L822 (2.3356, 1.8201) -> (2.3764, 1.7984)
  line L823 (2.3764, 1.7984) -> (2.4229, 1.7836)
  line L824 (2.4229, 1.7836) -> (2.4747, 1.776)
  line L825 (2.4747, 1.776) -> (2.531, 1.7761)
  line L826 (2.531, 1.7761) -> (2.5915, 1.7842)
  line L827 (2.5915, 1.7842) -> (2.6555, 1.8006)
  line L828 (2.6555, 1.8006) -> (2.7225, 1.8257)
  line L829 (2.7225, 1.8257) -> (2.7917, 1.8597)
  line L830 (2.7917, 1.8597) -> (2.8626, 1.9029)
  line L831 (2.8626, 1.9029) -> (2.9345, 1.9553)
  line L832 (2.9345, 1.9553) -> (3.0068, 2.0173)
  line L833 (3.0068, 2.0173) -> (3.0787, 2.0888)
  line L834 (3.0787, 2.0888) -> (3.1415, 2.1601)
  line L835 (3.1415, 2.1601) -> (3.2047, 2.186)
  line L836 (3.2047, 2.186) -> (3.2918, 2.2134)
  line L837 (3.2918, 2.2134) -> (3.4098, 2.2401)
  line L838 (3.4098, 2.2401) -> (3.5525, 2.2601)
  line L839 (3.5525, 2.2601) -> (3.6357, 2.2666)
  line L840 (3.6357, 2.2666) -> (3.7254, 2.2698)
  line L841 (3.7254, 2.2698) -> (3.8215, 2.2692)
  line L842 (3.8215, 2.2692) -> (3.9233, 2.2643)
  line L843 (3.9233, 2.2643) -> (4.0329, 2.2544)
  line L844 (4.0329, 2.2544) -> (4.1472, 2.2392)
  line L845 (4.1472, 2.2392) -> (4.2685, 2.2179)
  line L846 (4.2685, 2.2179) -> (4.3942, 2.1904)
  line L847 (4.3942, 2.1904) -> (4.509, 2.1603)
  arc A15 (4.7159, 1.6608) -> (4.509, 2.1603) centre (-0.0002, -0.0001) ccw
  line L848 (4.7159, 1.6608) -> (4.656, 1.5583)
  line L849 (4.656, 1.5583) -> (4.5866, 1.4499)
  line L850 (4.5866, 1.4499) -> (4.5159, 1.3491)
  line L851 (4.5159, 1.3491) -> (4.4458, 1.2575)
  line L852 (4.4458, 1.2575) -> (4.3753, 1.173)
  line L853 (4.3753, 1.173) -> (4.3068, 1.0976)
  line L854 (4.3068, 1.0976) -> (4.2393, 1.0292)
  line L855 (4.2393, 1.0292) -> (4.1736, 0.968)
  line L856 (4.1736, 0.968) -> (4.1102, 0.9138)
  line L857 (4.1102, 0.9138) -> (3.9952, 0.8271)
  line L858 (3.9952, 0.8271) -> (3.8928, 0.7625)
  line L859 (3.8928, 0.7625) -> (3.8118, 0.7203)
  line L860 (3.8118, 0.7203) -> (3.7488, 0.6939)
  line L861 (3.7488, 0.6939) -> (3.654, 0.6999)
  line L862 (3.654, 0.6999) -> (3.5526, 0.6996)
  line L863 (3.5526, 0.6996) -> (3.4577, 0.6923)
  line L864 (3.4577, 0.6923) -> (3.3697, 0.6786)
  line L865 (3.3697, 0.6786) -> (3.2891, 0.6589)
  line L866 (3.2891, 0.6589) -> (3.2161, 0.634)
  line L867 (3.2161, 0.634) -> (3.151, 0.6044)
  line L868 (3.151, 0.6044) -> (3.0941, 0.5708)
  line L869 (3.0941, 0.5708) -> (3.0456, 0.5338)
  line L870 (3.0456, 0.5338) -> (3.0057, 0.494)
  line L871 (3.0057, 0.494) -> (2.9745, 0.452)
  line L872 (2.9745, 0.452) -> (2.9521, 0.4086)
  line L873 (2.9521, 0.4086) -> (2.9385, 0.3645)
  line L874 (2.9385, 0.3645) -> (2.9338, 0.3147)
  line L875 (2.9338, 0.3147) -> (2.9482, 0.1004)
  line L876 (2.9482, 0.1004) -> (2.9499, -0.0001)
  line L877 (2.9499, -0.0001) -> (2.9482, -0.1006)
  line L878 (2.9482, -0.1006) -> (2.9338, -0.3148)
  line L879 (2.9338, -0.3148) -> (2.9385, -0.3646)
  line L880 (2.9385, -0.3646) -> (2.9521, -0.4088)
  line L881 (2.9521, -0.4088) -> (2.9745, -0.4522)
  line L882 (2.9745, -0.4522) -> (3.0057, -0.4941)
  line L883 (3.0057, -0.4941) -> (3.0456, -0.5339)
  line L884 (3.0456, -0.5339) -> (3.0941, -0.571)
  line L885 (3.0941, -0.571) -> (3.151, -0.6046)
  line L886 (3.151, -0.6046) -> (3.2161, -0.6342)
  line L887 (3.2161, -0.6342) -> (3.2891, -0.6591)
  line L888 (3.2891, -0.6591) -> (3.3697, -0.6787)
  line L889 (3.3697, -0.6787) -> (3.4577, -0.6925)
  line L890 (3.4577, -0.6925) -> (3.5526, -0.6998)
  line L891 (3.5526, -0.6998) -> (3.654, -0.7001)
  line L892 (3.654, -0.7001) -> (3.7488, -0.6941)
  line L893 (3.7488, -0.6941) -> (3.8118, -0.7205)
  line L894 (3.8118, -0.7205) -> (3.8928, -0.7626)
  line L895 (3.8928, -0.7626) -> (3.9952, -0.8272)
  line L896 (3.9952, -0.8272) -> (4.1102, -0.914)
  line L897 (4.1102, -0.914) -> (4.1736, -0.9682)
  line L898 (4.1736, -0.9682) -> (4.2393, -1.0294)
  line L899 (4.2393, -1.0294) -> (4.3068, -1.0977)
  line L900 (4.3068, -1.0977) -> (4.3753, -1.1732)
  line L901 (4.3753, -1.1732) -> (4.4458, -1.2577)
  line L902 (4.4458, -1.2577) -> (4.5159, -1.3492)
  line L903 (4.5159, -1.3492) -> (4.5866, -1.4501)
  line L904 (4.5866, -1.4501) -> (4.656, -1.5584)
  line L905 (4.656, -1.5584) -> (4.7159, -1.6609)
  arc A16 (4.509, -2.1604) -> (4.7159, -1.6609) centre (-0.0002, -0.0001) ccw
  line L906 (4.509, -2.1604) -> (4.3942, -2.1905)
  line L907 (4.3942, -2.1905) -> (4.2685, -2.2181)
  line L908 (4.2685, -2.2181) -> (4.1472, -2.2394)
  line L909 (4.1472, -2.2394) -> (4.0329, -2.2546)
  line L910 (4.0329, -2.2546) -> (3.9233, -2.2644)
  line L911 (3.9233, -2.2644) -> (3.8215, -2.2694)
  line L912 (3.8215, -2.2694) -> (3.7254, -2.27)
  line L913 (3.7254, -2.27) -> (3.6357, -2.2668)
  line L914 (3.6357, -2.2668) -> (3.5525, -2.2603)
  line L915 (3.5525, -2.2603) -> (3.4098, -2.2403)
  line L916 (3.4098, -2.2403) -> (3.2918, -2.2136)
  line L917 (3.2918, -2.2136) -> (3.2047, -2.1861)
  line L918 (3.2047, -2.1861) -> (3.1415, -2.1602)
  line L919 (3.1415, -2.1602) -> (3.0787, -2.089)
  line L920 (3.0787, -2.089) -> (3.0068, -2.0174)